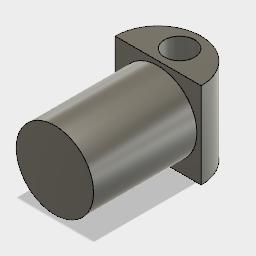
回転部 v7 (Autodesk Fusion 360 design; units mm, degrees)
Autodesk Fusion 360 part; units mm, degrees
sketch "スケッチ1" plane through (0, 0, 0) normal (0, 1, 0) x (1, 0, 0)
  line L0 (0, 5) -> (0, 5)
  line L1 (1.75, 0) -> (22.5, 0)
  line L2 (1.75, 0) -> (22.5, 0)
  line L3 (0, -1.75) -> (0, -22.5)
  arc A0 (5, -2.5) -> (-5, -2.5) centre (0, -2.5) ccw
  line L4 (-5, -2.5) -> (0, -2.5)
  line L5 (0, -2.5) -> (5, -2.5)
  dimension "d21" = 10
  measures "d21" distance of A0.end A0.start
extrude "押し出し1" add sketch "スケッチ1" along normal blind 10
sketch "スケッチ8" plane through (0, 10, 0) normal (0, 1, 0) x (-1, 0, 0)
  line L0 (5, 2.5) -> (-5, 2.5)
  arc A0 (-5, 2.5) -> (5, 2.5) centre (0, 2.5) ccw
  line L1 (-1.75, 0, -10) -> (-22.5, 0, -10)
  line L2 (0, 1.75, -10) -> (0, 22.5, -10)
  circle A1 centre (0, 0) radius 1.75
  dimension "d25" = 3.5
  measures "d25" diameter of A1
hole "穴1" at (0, 10, 0) direction (0, -1, 0) diameter 3.5 end through all
sketch "スケッチ10" plane through (0, 0, 2.5) normal (0, 0, 1) x (1, 0, 0)
  line L0 (5, 0) -> (5, 10)
  line L1 (5, 10) -> (-5, 10)
  line L2 (-5, 10) -> (-5, 0)
  arc A0 through (-5, 0, 0) (0, 0, -5) (5, 0, 0)
  line L3 (-5, 0) -> (-5, 10)
  arc A1 through (-5, 10, 0) (0, 10, -5) (5, 10, 0)
  line L4 (5, 10) -> (5, 0)
  line L5 (1.75, 0, -2.5) -> (22.5, 0, -2.5)
  line L6 (0, 0, -0.75) -> (0, 0, 20)
  line L7 (0, 1.75, -2.5) -> (0, 22.5, -2.5)
  circle A2 through (1.75, 0, -2.5) (-0.875, 0, -0.9845) (-0.875, 0, -4.0155)
  circle A3 through (-1.75, 10, -2.5) (0.875, 10, -0.9845) (0.875, 10, -4.0155)
  circle A4 centre (0, 5) radius 4.5
  line L8 (-5, 0) -> (5, 10) construction
  line L9 (-5, 10) -> (5, 0) construction
  dimension "d29" = 9
  measures "d29" diameter of A4
extrude "押し出し4" add sketch "スケッチ10" along normal blind 12
extrude "押し出し3" [rolled back] along distance 50 taper angle 0
